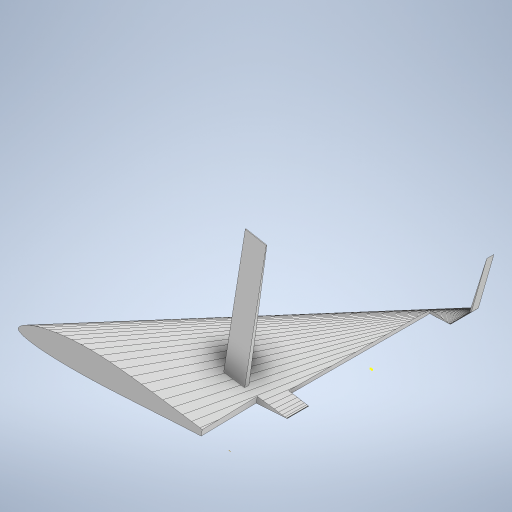
# Autodesk Inventor part: Część3
Saved by Autodesk Inventor 2023 (Build 270158000, 158)
## iProperties
Created: 2024-01-30
Part Number: Część3
Material: Ogólny
Document SubType Name: Modeling
Designer: domin
Density: 1 g/cm^3
Appearance: Domyślna
Author: domin
Autodesk Inventor part; units mm, degrees
ref_plane "YZ Plane" through (0, 0, 0) normal (1, 0, 0) x (0, 1, 0)
ref_plane "XZ Plane" through (0, 0, 0) normal (0, 1, 0) x (-1, 0, 0)
sketch "Szkic1" plane through (0, 0, 0) normal (0, 0, 1) x (1, 0, 0)
  line L0 (1, 0) -> (0.9965, 0.0005)
  line L1 (0.9965, 0.0005) -> (0.9863, 0.002)
  line L2 (0.9863, 0.002) -> (0.9701, 0.0049)
  line L3 (0.9701, 0.0049) -> (0.9487, 0.0088)
  line L4 (0.9487, 0.0088) -> (0.9224, 0.0134)
  line L5 (0.9224, 0.0134) -> (0.8913, 0.0184)
  line L6 (0.8913, 0.0184) -> (0.8558, 0.024)
  line L7 (0.8558, 0.024) -> (0.8163, 0.0301)
  line L8 (0.8163, 0.0301) -> (0.7736, 0.0367)
  line L9 (0.7736, 0.0367) -> (0.7281, 0.0435)
  line L10 (0.7281, 0.0435) -> (0.6804, 0.0506)
  line L11 (0.6804, 0.0506) -> (0.6313, 0.0576)
  line L12 (0.6313, 0.0576) -> (0.5814, 0.0644)
  line L13 (0.5814, 0.0644) -> (0.5313, 0.0708)
  line L14 (0.5313, 0.0708) -> (0.4817, 0.0764)
  line L15 (0.4817, 0.0764) -> (0.4331, 0.0808)
  line L16 (0.4331, 0.0808) -> (0.3857, 0.0836)
  line L17 (0.3857, 0.0836) -> (0.3398, 0.0848)
  line L18 (0.3398, 0.0848) -> (0.2957, 0.0843)
  line L19 (0.2957, 0.0843) -> (0.2536, 0.0821)
  line L20 (0.2536, 0.0821) -> (0.2137, 0.0782)
  line L21 (0.2137, 0.0782) -> (0.1762, 0.073)
  line L22 (0.1762, 0.073) -> (0.1416, 0.0667)
  line L23 (0.1416, 0.0667) -> (0.1102, 0.0594)
  line L24 (0.1102, 0.0594) -> (0.0823, 0.0514)
  line L25 (0.0823, 0.0514) -> (0.0581, 0.0428)
  line L26 (0.0581, 0.0428) -> (0.0379, 0.0338)
  line L27 (0.0379, 0.0338) -> (0.0219, 0.0247)
  line L28 (0.0219, 0.0247) -> (0.0102, 0.0157)
  line L29 (0.0102, 0.0157) -> (0.0028, 0.0071)
  line L30 (0.0028, 0.0071) -> (0, -0.0001)
  line L31 (0, -0.0001) -> (0.003, -0.0063)
  line L32 (0.003, -0.0063) -> (0.0121, -0.012)
  line L33 (0.0121, -0.012) -> (0.0263, -0.0175)
  line L34 (0.0263, -0.0175) -> (0.0454, -0.0223)
  line L35 (0.0454, -0.0223) -> (0.0694, -0.0265)
  line L36 (0.0694, -0.0265) -> (0.0981, -0.0299)
  line L37 (0.0981, -0.0299) -> (0.1311, -0.0326)
  line L38 (0.1311, -0.0326) -> (0.1682, -0.0345)
  line L39 (0.1682, -0.0345) -> (0.2089, -0.0357)
  line L40 (0.2089, -0.0357) -> (0.2529, -0.0361)
  line L41 (0.2529, -0.0361) -> (0.2997, -0.0359)
  line L42 (0.2997, -0.0359) -> (0.3486, -0.0349)
  line L43 (0.3486, -0.0349) -> (0.3994, -0.033)
  line L44 (0.3994, -0.033) -> (0.4517, -0.0304)
  line L45 (0.4517, -0.0304) -> (0.505, -0.0274)
  line L46 (0.505, -0.0274) -> (0.5586, -0.0243)
  line L47 (0.5586, -0.0243) -> (0.6119, -0.021)
  line L48 (0.6119, -0.021) -> (0.6641, -0.0179)
  line L49 (0.6641, -0.0179) -> (0.7147, -0.0149)
  line L50 (0.7147, -0.0149) -> (0.7628, -0.0121)
  line L51 (0.7628, -0.0121) -> (0.808, -0.0096)
  line L52 (0.808, -0.0096) -> (0.8495, -0.0074)
  line L53 (0.8495, -0.0074) -> (0.8868, -0.0056)
  line L54 (0.8868, -0.0056) -> (0.9194, -0.0039)
  line L55 (0.9194, -0.0039) -> (0.947, -0.0024)
  line L56 (0.947, -0.0024) -> (0.9693, -0.0011)
  line L57 (0.9693, -0.0011) -> (0.986, -0.0003)
  line L58 (0.986, -0.0003) -> (0.9964, 0)
  line L59 (0.9964, 0) -> (1, 0)
  point P0 (0, 0)
  dimension "d0" = 7.265
  dimension "d1" = 178.531
  dimension "d2" = 8.69
  dimension "d3" = 177.182
  dimension "d4" = 169.921
  dimension "d5" = 176.889
  dimension "d6" = 169.375
  dimension "d7" = 2.564
  dimension "d8" = 169.6
  dimension "d9" = 1.94
  dimension "d10" = 10.161
  dimension "d11" = 1.679
  dimension "d12" = 10.163
  dimension "d13" = 1.544
  dimension "d14" = 169.716
  dimension "d15" = 1.444
  dimension "d16" = 169.577
  dimension "d17" = 1.307
  dimension "d18" = 169.455
  dimension "d19" = 1.131
  dimension "d20" = 169.349
  dimension "d21" = 0.893
  dimension "d22" = 169.285
  dimension "d23" = 0.513
  dimension "d24" = 169.267
  dimension "d25" = 0.008
  dimension "d26" = 169.332
  dimension "d27" = 0.835
  dimension "d28" = 169.514
  dimension "d29" = 2.13
  dimension "d30" = 10.09
  dimension "d31" = 3.799
  dimension "d32" = 9.352
  dimension "d33" = 5.753
  dimension "d34" = 8.423
  dimension "d35" = 172.046
  dimension "d36" = 7.571
  dimension "d37" = 169.676
  dimension "d38" = 167.212
  dimension "d39" = 6.666
  dimension "d40" = 164.847
  dimension "d41" = 5.621
  dimension "d42" = 162.409
  dimension "d43" = 4.316
  dimension "d44" = 159.75
  dimension "d45" = 2.659
  dimension "d46" = 156.733
  dimension "d47" = 0.455
  dimension "d48" = 153.128
  dimension "d49" = 2.546
  dimension "d50" = 148.712
  dimension "d51" = 6.919
  dimension "d52" = 143.002
  dimension "d53" = 13.822
  dimension "d54" = 135.169
  dimension "d55" = 25.215
  dimension "d56" = 123.591
  dimension "d57" = 56.283
  dimension "d58" = 103.678
  dimension "d59" = 0.1265
  dimension "d60" = 0
  dimension "d61" = 0.1517
  dimension "d62" = 0.0248
  dimension "d63" = 0.1746
  constraints: 120 end point, 1 horizontal
  measures "d0" angle of L0 L59
  measures "d1" angle of L0 L1
  measures "d2" angle of L0 L58
  measures "d3" angle of L0 L2
  measures "d4" angle of L0 L57
  measures "d5" angle of L0 L3
  measures "d6" angle of L0 L56
  measures "d7" angle of L0 L4
  measures "d8" angle of L0 L55
  measures "d9" angle of L0 L5
  measures "d10" angle of L0 L54
  measures "d11" angle of L0 L6
  measures "d12" angle of L0 L53
  measures "d13" angle of L0 L7
  measures "d14" angle of L0 L52
  measures "d15" angle of L0 L8
  measures "d16" angle of L0 L51
  measures "d17" angle of L0 L9
  measures "d18" angle of L0 L50
  measures "d19" angle of L0 L10
  measures "d20" angle of L0 L49
  measures "d21" angle of L0 L11
  measures "d22" angle of L0 L48
  measures "d23" angle of L0 L12
  measures "d24" angle of L0 L47
  measures "d25" angle of L0 L13
  measures "d26" angle of L0 L46
  measures "d27" angle of L0 L14
  measures "d28" angle of L0 L45
  measures "d29" angle of L0 L15
  measures "d30" angle of L0 L44
  measures "d31" angle of L0 L16
  measures "d32" angle of L0 L43
  measures "d33" angle of L0 L17
  measures "d34" angle of L0 L42
  measures "d35" angle of L0 L18
  measures "d36" angle of L0 L41
  measures "d37" angle of L0 L19
  measures "d38" angle of L0 L20
  measures "d39" angle of L0 L40
  measures "d40" angle of L0 L21
  measures "d41" angle of L0 L39
  measures "d42" angle of L0 L22
  measures "d43" angle of L0 L38
  measures "d44" angle of L0 L23
  measures "d45" angle of L0 L37
  measures "d46" angle of L0 L24
  measures "d47" angle of L0 L36
  measures "d48" angle of L0 L25
  measures "d49" angle of L0 L35
  measures "d50" angle of L0 L26
  measures "d51" angle of L0 L34
  measures "d52" angle of L0 L27
  measures "d53" angle of L0 L33
  measures "d54" angle of L0 L28
  measures "d55" angle of L0 L32
  measures "d56" angle of L0 L29
  measures "d57" angle of L0 L31
  measures "d58" angle of L0 L30
  measures "d59" distance from line of point (0, 0) L0
  measures "d60" distance from line of point (0, 0) L59
  measures "d61" distance from line of point (0, 0) L1
  measures "d62" distance from line of point (0, 0) L58
  measures "d63" distance from line of point (0, 0) L2
ref_plane "Płaszczyzna konstrukcyjna2" through (0, 0, 175) normal (0, 0, 1) x (1, 0, 0)
sketch "Szkic6" plane through (0, 0, 175) normal (0, 0, 1) x (1, 0, 0)
  line L0 (1, 0) -> (0.4705, 0.0675)
  line L1 (0.4705, 0.0675) -> (-1.0625, 0.303)
  line L2 (-1.0625, 0.303) -> (-3.4835, 0.7335)
  line L3 (-3.4835, 0.7335) -> (-6.695, 1.3215)
  line L4 (-6.695, 1.3215) -> (-10.643, 2.0055)
  line L5 (-10.643, 2.0055) -> (-15.308, 2.7615)
  line L6 (-15.308, 2.7615) -> (-20.636, 3.6)
  line L7 (-20.636, 3.6) -> (-26.5505, 4.5165)
  line L8 (-26.5505, 4.5165) -> (-32.9645, 5.499)
  line L9 (-32.9645, 5.499) -> (-39.791, 6.528)
  line L10 (-39.791, 6.528) -> (-46.9355, 7.5825)
  line L11 (-46.9355, 7.5825) -> (-54.302, 8.6385)
  line L12 (-54.302, 8.6385) -> (-61.7915, 9.6615)
  line L13 (-61.7915, 9.6615) -> (-69.3065, 10.6185)
  line L14 (-69.3065, 10.6185) -> (-76.7465, 11.457)
  line L15 (-76.7465, 11.457) -> (-84.041, 12.1125)
  line L16 (-84.041, 12.1125) -> (-91.1495, 12.543)
  line L17 (-91.1495, 12.543) -> (-98.0285, 12.7245)
  line L18 (-98.0285, 12.7245) -> (-104.6405, 12.645)
  line L19 (-104.6405, 12.645) -> (-110.9555, 12.3075)
  line L20 (-110.9555, 12.3075) -> (-116.9435, 11.7285)
  line L21 (-116.9435, 11.7285) -> (-122.5625, 10.95)
  line L22 (-122.5625, 10.95) -> (-127.757, 10.0035)
  line L23 (-127.757, 10.0035) -> (-132.473, 8.916)
  line L24 (-132.473, 8.916) -> (-136.6625, 7.7145)
  line L25 (-136.6625, 7.7145) -> (-140.288, 6.423)
  line L26 (-140.288, 6.423) -> (-143.3135, 5.0745)
  line L27 (-143.3135, 5.0745) -> (-145.7165, 3.702)
  line L28 (-145.7165, 3.702) -> (-147.4775, 2.3475)
  line L29 (-147.4775, 2.3475) -> (-148.5815, 1.071)
  line L30 (-148.5815, 1.071) -> (-149, -0.0225)
  line L31 (-149, -0.0225) -> (-148.544, -0.939)
  line L32 (-148.544, -0.939) -> (-147.182, -1.806)
  line L33 (-147.182, -1.806) -> (-145.058, -2.625)
  line L34 (-145.058, -2.625) -> (-142.1855, -3.351)
  line L35 (-142.1855, -3.351) -> (-138.5855, -3.9735)
  line L36 (-138.5855, -3.9735) -> (-134.2895, -4.4865)
  line L37 (-134.2895, -4.4865) -> (-129.3365, -4.8855)
  line L38 (-129.3365, -4.8855) -> (-123.7745, -5.172)
  line L39 (-123.7745, -5.172) -> (-117.6605, -5.3475)
  line L40 (-117.6605, -5.3475) -> (-111.062, -5.4165)
  line L41 (-111.062, -5.4165) -> (-104.051, -5.379)
  line L42 (-104.051, -5.379) -> (-96.7085, -5.2305)
  line L43 (-96.7085, -5.2305) -> (-89.0945, -4.953)
  line L44 (-89.0945, -4.953) -> (-81.2525, -4.566)
  line L45 (-81.2525, -4.566) -> (-73.2575, -4.116)
  line L46 (-73.2575, -4.116) -> (-65.21, -3.6375)
  line L47 (-65.21, -3.6375) -> (-57.2165, -3.153)
  line L48 (-57.2165, -3.153) -> (-49.379, -2.6805)
  line L49 (-49.379, -2.6805) -> (-41.7995, -2.232)
  line L50 (-41.7995, -2.232) -> (-34.5755, -1.818)
  line L51 (-34.5755, -1.818) -> (-27.806, -1.4445)
  line L52 (-27.806, -1.4445) -> (-21.578, -1.116)
  line L53 (-21.578, -1.116) -> (-15.9785, -0.8325)
  line L54 (-15.9785, -0.8325) -> (-11.087, -0.585)
  line L55 (-11.087, -0.585) -> (-6.9515, -0.3585)
  line L56 (-6.9515, -0.3585) -> (-3.605, -0.162)
  line L57 (-3.605, -0.162) -> (-1.103, -0.039)
  line L58 (-1.103, -0.039) -> (0.4645, 0)
  line L59 (0.4645, 0) -> (1, 0)
  point P0 (0, 0)
  dimension "d367" = 7.265
  dimension "d368" = 178.531
  dimension "d369" = 8.69
  dimension "d370" = 177.182
  dimension "d371" = 169.921
  dimension "d372" = 176.889
  dimension "d373" = 169.375
  dimension "d374" = 2.564
  dimension "d375" = 169.6
  dimension "d376" = 1.94
  dimension "d377" = 10.161
  dimension "d378" = 1.679
  dimension "d379" = 10.163
  dimension "d380" = 1.544
  dimension "d381" = 169.716
  dimension "d382" = 1.444
  dimension "d383" = 169.577
  dimension "d384" = 1.307
  dimension "d385" = 169.455
  dimension "d386" = 1.131
  dimension "d387" = 169.349
  dimension "d388" = 0.893
  dimension "d389" = 169.285
  dimension "d390" = 0.513
  dimension "d391" = 169.267
  dimension "d392" = 0.008
  dimension "d393" = 169.332
  dimension "d394" = 0.835
  dimension "d395" = 169.514
  dimension "d396" = 2.13
  dimension "d397" = 10.09
  dimension "d398" = 3.799
  dimension "d399" = 9.352
  dimension "d400" = 5.753
  dimension "d401" = 8.423
  dimension "d402" = 172.046
  dimension "d403" = 7.571
  dimension "d404" = 169.676
  dimension "d405" = 167.212
  dimension "d406" = 6.666
  dimension "d407" = 164.847
  dimension "d408" = 5.621
  dimension "d409" = 162.409
  dimension "d410" = 4.316
  dimension "d411" = 159.75
  dimension "d412" = 2.659
  dimension "d413" = 156.733
  dimension "d414" = 0.455
  dimension "d415" = 153.128
  dimension "d416" = 2.546
  dimension "d417" = 148.712
  dimension "d418" = 6.919
  dimension "d419" = 143.002
  dimension "d420" = 13.822
  dimension "d421" = 135.169
  dimension "d422" = 25.215
  dimension "d423" = 123.591
  dimension "d424" = 56.283
  dimension "d425" = 103.678
  dimension "d426" = 0.1265
  dimension "d427" = 0
  dimension "d428" = 0.1382
  dimension "d429" = 0.0115
  dimension "d430" = 0.1123
  constraints: 120 end point, 1 horizontal
  measures "d367" angle of L0 L59
  measures "d368" angle of L0 L1
  measures "d369" angle of L0 L58
  measures "d370" angle of L0 L2
  measures "d371" angle of L0 L57
  measures "d372" angle of L0 L3
  measures "d373" angle of L0 L56
  measures "d374" angle of L0 L4
  measures "d375" angle of L0 L55
  measures "d376" angle of L0 L5
  measures "d377" angle of L0 L54
  measures "d378" angle of L0 L6
  measures "d379" angle of L0 L53
  measures "d380" angle of L0 L7
  measures "d381" angle of L0 L52
  measures "d382" angle of L0 L8
  measures "d383" angle of L0 L51
  measures "d384" angle of L0 L9
  measures "d385" angle of L0 L50
  measures "d386" angle of L0 L10
  measures "d387" angle of L0 L49
  measures "d388" angle of L0 L11
  measures "d389" angle of L0 L48
  measures "d390" angle of L0 L12
  measures "d391" angle of L0 L47
  measures "d392" angle of L0 L13
  measures "d393" angle of L0 L46
  measures "d394" angle of L0 L14
  measures "d395" angle of L0 L45
  measures "d396" angle of L0 L15
  measures "d397" angle of L0 L44
  measures "d398" angle of L0 L16
  measures "d399" angle of L0 L43
  measures "d400" angle of L0 L17
  measures "d401" angle of L0 L42
  measures "d402" angle of L0 L18
  measures "d403" angle of L0 L41
  measures "d404" angle of L0 L19
  measures "d405" angle of L0 L20
  measures "d406" angle of L0 L40
  measures "d407" angle of L0 L21
  measures "d408" angle of L0 L39
  measures "d409" angle of L0 L22
  measures "d410" angle of L0 L38
  measures "d411" angle of L0 L23
  measures "d412" angle of L0 L37
  measures "d413" angle of L0 L24
  measures "d414" angle of L0 L36
  measures "d415" angle of L0 L25
  measures "d416" angle of L0 L35
  measures "d417" angle of L0 L26
  measures "d418" angle of L0 L34
  measures "d419" angle of L0 L27
  measures "d420" angle of L0 L33
  measures "d421" angle of L0 L28
  measures "d422" angle of L0 L32
  measures "d423" angle of L0 L29
  measures "d424" angle of L0 L31
  measures "d425" angle of L0 L30
  measures "d426" distance from line of point (0, 0) L0
  measures "d427" distance from line of point (0, 0) L59
  measures "d428" distance from line of point (0, 0) L1
  measures "d429" distance from line of point (0, 0) L58
  measures "d430" distance from line of point (0, 0) L2
loft "Wyciągnięcie złożone2" add profiles "Szkic1", "Szkic6"
ref_plane "Płaszczyzna konstrukcyjna3" through (0.4817, 0.0764, 0) normal (0.1803699, 0.9834745, 0.0156405) x (-0.4030251, 0.0593912, 0.9132598)
sketch "Szkic7" plane through (0.4817, 0.0764, 0) normal (0.1803699, 0.9834745, 0.0156405) x (-0.4030251, 0.0593912, 0.9132598)
  point P0 (0.1896, -0.4191)
sketch "Szkic8" plane through (0.4817, 0.0764, 0) normal (0.1803699, 0.9834745, 0.0156405) x (-0.4030251, 0.0593912, 0.9132598)
  line L0 (-0.2134, 0.4781) -> (159.607, 71.7166) projected
  line L1 (159.2965, 72.4134) -> (123.0788, 55.4345)
  line L2 (123.0788, 55.4345) -> (131.9754, 36.4571)
  line L3 (131.9754, 36.4571) -> (168.1931, 53.436)
  line L4 (168.1931, 53.436) -> (159.2965, 72.4134)
  point P0 (0.1896, -0.4191)
  dimension "d493" = 40
  dimension "d494" = 91.093
  dimension "d495" = 20.9593
  dimension "d496" = 0.0146
  constraints: 8 end point, 2 parallel, 1 perpendicular, 1 point on line
  measures "d493" distance of L1.start L1.end
  measures "d494" angle of L4 L0
  measures "d495" distance between parallel lines of L1 L3
  measures "d496" distance from line of L0.end L4
extrude "Wyciągnięcie proste2" cut sketch "Szkic8" along normal blind 40 and the other way blind 5
sketch "Szkic9" plane through (0.4817, 0.0764, 0) normal (0.1803699, 0.9834745, 0.0156405) x (-0.4030251, 0.0593912, 0.9132598)
  line L0 (-0.2078, 0.4656) -> (123.7554, 53.9912) projected
  line L1 (109.2926, 48.8774) -> (17.9018, 8.2851)
  line L2 (17.9018, 8.2851) -> (23.5848, -4.5096)
  line L3 (23.5848, -4.5096) -> (114.9755, 36.0826)
  line L4 (114.9755, 36.0826) -> (109.2926, 48.8774)
  line L5 (-0.2078, 0.4654) -> (123.1603, 55.2608) projected
  point P0 (0.1896, -0.4191)
  dimension "d501" = 100
  dimension "d502" = 14
  dimension "d503" = 14.2047
  constraints: 8 end point, 3 parallel, 1 perpendicular, 1 point on line
  measures "d501" distance of L1.start L1.end
  measures "d502" distance of L2.end L1.end
  measures "d503" distance between parallel lines of L3 L5
extrude "Wyciągnięcie proste3" cut sketch "Szkic9" along normal mid plane 40
sketch "Szkic10" plane through (0.7505, -0.0046, 19.726) normal (-0.9835902, 0.1804121, -0.001318) x (-0.0013322, 0.0000425, 0.9999991)
  line L0 (-0.001, -1.2787) -> (-0.001, 2.7279)
  line L1 (-0.001, 2.7279) -> (100.0156, 2.7279)
  line L2 (100.0156, 2.7279) -> (100.0156, -1.2787)
  line L3 (100.0156, -1.2787) -> (-0.001, -1.2787)
  point P0 (-19.725, -0.1348)
  dimension "d506" = 100.0167
  dimension "d507" = 4.0066
  dimension "d508" = 119.7406
  dimension "d509" = 2.8627
  constraints: 8 end point, 2 parallel, 1 perpendicular, 1 vertical
  measures "d506" distance between parallel lines of L0 L2
  measures "d507" distance between parallel lines of L1 L3
  measures "d508" distance from line of point (-19.725, -0.135) L2
  measures "d509" distance from line of point (-19.725, -0.135) L1
extrude "Wyciągnięcie proste4" cut sketch "Szkic10" against normal blind 40
sketch "Szkic11" plane through (0.4817, 0.0764, 0) normal (0.1803699, 0.9834745, 0.0156405) x (-0.4030251, 0.0593912, 0.9132598)
  line L0 (135.9854, 29.0374) -> (142.0529, 15.3193)
  line L1 (142.0529, 15.3193) -> (139.2712, 14.089)
  line L2 (139.2712, 14.089) -> (133.2037, 27.8071)
  line L3 (133.2037, 27.8071) -> (135.9854, 29.0374)
  line L4 (109.2944, 48.8805) -> (123.2563, 55.0559) projected
  point P0 (0.1896, -0.4191)
  dimension "d512" = 15
  dimension "d513" = 43.9438
  dimension "d514" = 3.0416
  dimension "d515" = 1.1167
  constraints: 8 end point, 3 parallel, 1 perpendicular
  measures "d512" distance of L0.start L0.end
  measures "d513" distance between parallel lines of L1 L4
  measures "d514" distance between parallel lines of L2 L0
  measures "d515" distance from line of L4.end L0
ref_plane "Płaszczyzna konstrukcyjna4" through (14.9113, 78.7543, 1.2512) normal (0.1803699, 0.9834745, 0.0156405) x (-0.4030251, 0.0593912, 0.9132598)
sketch "Szkic12" plane through (14.9113, 78.7543, 1.2512) normal (0.1803699, 0.9834745, 0.0156405) x (-0.4030251, 0.0593912, 0.9132598)
  line L0 (127.0023, 9.6411) -> (133.116, -4.0564)
  line L1 (133.116, -4.0564) -> (132.6594, -4.2602)
  line L2 (132.6594, -4.2602) -> (126.5457, 9.4374)
  line L3 (126.5457, 9.4374) -> (127.0023, 9.6411)
  line L4 (173.6222, 40.3019) -> (176.4345, 34.0009) projected
  point P0 (0.1896, -0.4191)
  dimension "d517" = 15
  dimension "d518" = 0.5
  dimension "d519" = 55.0686
  dimension "d520" = 17.0969
  constraints: 8 end point, 3 parallel, 1 perpendicular
  measures "d517" distance of L0.start L0.end
  measures "d518" distance of L0.end L1.end
  measures "d519" distance between parallel lines of L0 L4
  measures "d520" distance from line of L4.end L1
loft "Wyciągnięcie złożone3" add profiles "Szkic11", "Szkic12"
ref_plane "Płaszczyzna konstrukcyjna5" through (-73.2575, -4.116, 75) normal (0, 0, 1) x (0.998237, 0.0593546, 0)
sketch "Szkic13" plane through (-73.2575, -4.116, 75) normal (0, 0, 1) x (0.998237, 0.0593546, 0)
  point P0 (74.3709, -0.2988)
  point P1 (73.3726, -0.2396)
sketch "Szkic14" plane through (0.5586, -0.0243, 0) normal (0, 0, -1) x (-0.998237, -0.0593546, 0)
  line L0 (-0.4421, -0.002) -> (-0.0288, 0.0226) projected
  line L1 (-0.4421, -0.002) -> (-13.7476, 37.7202)
  line L2 (-13.7476, 37.7202) -> (0.5562, 0.0574)
  line L3 (0.5562, 0.0574) -> (-0.4421, -0.002)
  point P0 (-0.0288, 0.0226)
  dimension "d529" = 40
  dimension "d530" = 72.607
  constraints: 6 end point
  measures "d529" distance of L0.start L1.end
  measures "d530" angle of L0 L2
extrude "Wyciągnięcie proste5" add sketch "Szkic14" against normal blind 5
